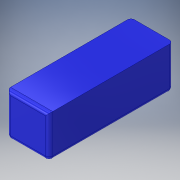
# Autodesk Inventor part: G5_50C_4S_2500mah_LiPo
Saved by Autodesk Inventor 2018 (Build 220112000, 112)
## iProperties
Created: 2017-09-19
Part Number: G5_50C_4S_2500mah_LiPo
Material: Generic
Document SubType Name: Modeling
Designer: snipe
Density: 1 g/cm^3
Appearance: Blue - Wall Paint - Glossy
Author: snipe
Autodesk Inventor part; units mm, degrees
ref_plane "YZ Plane" through (0, 0, 0) normal (1, 0, 0) x (0, 1, 0)
ref_plane "XZ Plane" through (0, 0, 0) normal (0, 1, 0) x (-1, 0, 0)
ref_plane "XY Plane" through (0, 0, 0) normal (0, 0, 1) x (1, 0, 0)
sketch "Sketch1" plane through (0, 0, 0) normal (0, 1, 0) x (-1, 0, 0)
  line L0 (0, -74.2) -> (0, 74.2) projected
  line L1 (-25.2, 0) -> (25.2, 0) projected
  line L2 (25.2, 0) -> (-25.2, 0) projected
  line L3 (0, -74.2) -> (0, 74.2) projected
  line L4 (18, -53) -> (-18, -53)
  line L5 (-18, -53) -> (-18, 53)
  line L6 (-18, 53) -> (18, 53)
  line L7 (18, 53) -> (18, -53)
  point P0 (0, 0)
  dimension "d0" = 36
  dimension "d1" = 106
  constraints: 8 end point, 2 parallel, 1 horizontal, 1 perpendicular, 2 other
  measures "d0" distance of L5.end L6.end
  measures "d1" distance of L4.end L5.end
extrude "Extrusion1" add sketch "Sketch1" along normal blind 36
fillet "Fillet1" radius 3.175 9 edges at (0, 36, 53) (0, 0, 53) (18, 0, 0) (-18, 0, 0) (-18, 18, 53) (18, 18, 53) (0, 0, -53) (-18, 18, -53) (18, 18, -53)
body "Solid1"
